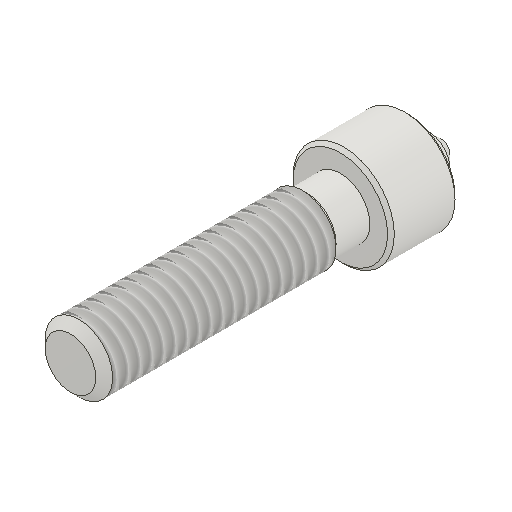
# Autodesk Inventor part: GRJ-03-119
Saved by Autodesk Inventor 2026.1 (Build 301233000, 233)
## iProperties
Company: Gree
Created: 2025-08-15
Part Number: GRJ-03-119
Material: Aço SAE 1045
Document SubType Name: Modeling
Designer: Willian Pinheiro
Density: 7.85 g/cm^3
Appearance: Aço
Mass: 2.46306 g
Surface Area: 3.36835 cm^2
Volume: 0.313766 cm^3
Description: Pino Suporte IPM
Project: GRJ-03
Checked By: Antonio Lucas
Engr Approved By: Antonio Lucas
Mfg Approved By: Anderson Oliveira
Dimensões: Ø6 x 22 mm
Total: 5
Author: Willian Pinheiro
Title: Soldagem
Revision Number: 00
Autodesk Inventor part; units mm, degrees
ref_plane "YZ Plane" through (0, 0, 0) normal (1, 0, 0) x (0, 1, 0)
ref_plane "XZ Plane" through (0, 0, 0) normal (0, 1, 0) x (-1, 0, 0)
ref_plane "XY Plane" through (0, 0, 0) normal (0, 0, 1) x (1, 0, 0)
sketch "Esboço1" plane through (0, 0, 0) normal (0, 0, 1) x (1, 0, 0)
  line L0 (0, -20.4) -> (0, 10.4) construction
  line L1 (-3.6, 0) -> (0.6, 0) construction
  line L2 (0, -16) -> (-2, -16)
  line L3 (-2, -16) -> (-2, 0)
  line L4 (-2, 0) -> (-3, 0)
  line L5 (-3, 0) -> (-3, 4)
  line L6 (-3, 4) -> (-1.25, 4)
  line L7 (-1.25, 4) -> (-1.25, 6)
  line L8 (-1.25, 6) -> (0, 6)
  line L9 (0, 6) -> (0, -16)
  line L10 (-0.5, 6) -> (-1.25, 5.25)
  line L11 (-2, -15.5) -> (-1.5, -16)
  line L12 (-3, 3.8) -> (-2.8, 4)
  line L13 (-3, 2) -> (0, 2) construction
  line L14 (-3, 0.2) -> (-2.8, 0)
  line L15 (-2, -2) -> (-1.75, -2)
  line L16 (-1.75, -2) -> (-1.75, 0)
  line L17 (-1.75, 0) -> (-2, 0)
  line L18 (-2, 0) -> (-2, -2)
  line L19 (-1.75, -2) -> (-2, -2.25)
  point P0 (0, 0)
  dimension "d0" = 2
  dimension "d1" = 6
  dimension "d2" = 2.5
  dimension "d3" = 0.75
  dimension "d4" = 0.75
  dimension "d5" = 4
  dimension "d6" = 16
  dimension "d7" = 22
  dimension "d8" = 4
  dimension "d9" = 0.5
  dimension "d10" = 0.5
  dimension "d12" = 0.2
  dimension "d13" = 0.2
  dimension "d16" = 3.5
  dimension "d17" = 2
  dimension "d18" = 0.25
  dimension "d19" = 0.25
  constraints: 36 end point, 12 point on line, 7 perpendicular, 2 horizontal, 2 parallel, 2 symmetric about line, 2 vertical, 1 collinear, 1 midpoint
  measures "d0" distance of L6.end L7.end
  measures "d1" diameter of L5 L0
  measures "d2" diameter of L7 L0
  measures "d3" horizontal distance of L10.start L10.end
  measures "d4" horizontal distance of L10.start L10.end
  measures "d5" distance between parallel lines of L4 L6
  measures "d6" distance between parallel lines of L2 L4
  measures "d7" distance between parallel lines of L2 L8
  measures "d8" diameter of L3 L0
  measures "d9" horizontal distance of L11.start L11.end
  measures "d10" horizontal distance of L11.start L11.end
  measures "d12" horizontal distance of L12.start L12.end
  measures "d13" horizontal distance of L12.start L12.end
  measures "d16" diameter of L16 L0
  measures "d17" distance between parallel lines of L4 L15
  measures "d18" horizontal distance of L15.end L19.end
  measures "d19" distance of L15.start L15.end
revolve "Revolução1" add sketch "Esboço1" angle 360 about axis through (0, -10, 0) along (0, 1, 0) contours L2 L11 L3 L19 L16 L17 L4 L14 L5 L12 L6 L7 L10 L8 L9
thread "Rosca1" size "M4x0.7" class "6g" standard "ISO Metric profile" full length
equation "\"d4\" = d3"
equation "\"d10\" = d9"
equation "\"d18\" = d19"
